Autodesk Inventor part; units mm, degrees
(part 10 of 10)
  spline S24 degree 5 poles (-3.4199, 4.4832) (-3.4186, 4.4814) (-3.4221, 4.4861) (-3.4215, 4.4854) (-3.4253, 4.4909) (-3.428, 4.4951) (-3.4307, 4.4992) (-3.4365, 4.5085) (-3.4424, 4.5184) (-3.4458, 4.5243) (-3.4538, 4.5385) (-3.4613, 4.5527) (-3.4656, 4.5609) (-3.4749, 4.5792) (-3.4837, 4.5978) (-3.4884, 4.608) (-3.4985, 4.6304) (-3.508, 4.6531) (-3.513, 4.6653) (-3.5233, 4.6916) (-3.5331, 4.7182) (-3.5382, 4.7323) (-3.5485, 4.7624) (-3.5582, 4.7926) (-3.5631, 4.8086) (-3.573, 4.8422) (-3.5823, 4.8761) (-3.587, 4.8938) (-3.5964, 4.9308) (-3.6049, 4.9679) (-3.6092, 4.9872) (-3.6176, 5.0274) (-3.6253, 5.0677) (-3.629, 5.0885) (-3.6363, 5.1317) (-3.6427, 5.175) (-3.6458, 5.1973) (-3.6518, 5.2433) (-3.6568, 5.2893) (-3.6592, 5.313) (-3.6636, 5.3617) (-3.667, 5.4104) (-3.6686, 5.4354) (-3.6712, 5.4865) (-3.673, 5.5377) (-3.6736, 5.5639) (-3.6744, 5.6173) (-3.6742, 5.6708) (-3.6739, 5.6981) (-3.6729, 5.7437) (-3.6712, 5.7892) (-3.6704, 5.8075) (-3.6696, 5.8257) (-3.6686, 5.8439) knots 0 0 0 0 0 0 0.005206 0.005206 0.005206 0.020768 0.020768 0.020768 0.045447 0.045447 0.045447 0.078301 0.078301 0.078301 0.118594 0.118594 0.118594 0.165744 0.165744 0.165744 0.219295 0.219295 0.219295 0.278897 0.278897 0.278897 0.344176 0.344176 0.344176 0.414704 0.414704 0.414704 0.490245 0.490245 0.490245 0.570535 0.570535 0.570535 0.655343 0.655343 0.655343 0.744467 0.744467 0.744467 0.837726 0.837726 0.837726 0.934962 0.934962 0.934962 1 1 1 1 1 1
  spline S25 degree 5 poles (-3.2267, 6.0991) (-3.2141, 6.0927) (-3.2016, 6.0863) (-3.1891, 6.0798) (-3.1559, 6.0624) (-3.123, 6.0445) (-3.1024, 6.0333) (-3.0623, 6.0108) (-3.0225, 5.9876) (-3.003, 5.9761) (-2.965, 5.9532) (-2.9273, 5.9297) (-2.9089, 5.9181) (-2.873, 5.8949) (-2.8375, 5.8711) (-2.8201, 5.8593) (-2.7864, 5.836) (-2.7531, 5.8121) (-2.7369, 5.8003) (-2.7054, 5.777) (-2.6743, 5.7531) (-2.6593, 5.7413) (-2.63, 5.7181) (-2.6012, 5.6945) (-2.5873, 5.6828) (-2.5603, 5.6599) (-2.5338, 5.6366) (-2.521, 5.6251) (-2.4964, 5.6027) (-2.4721, 5.5799) (-2.4605, 5.5688) (-2.4382, 5.547) (-2.4164, 5.5249) (-2.4059, 5.5142) (-2.386, 5.4933) (-2.3665, 5.472) (-2.3572, 5.4618) (-2.3396, 5.442) (-2.3223, 5.4218) (-2.3142, 5.4122) (-2.299, 5.3937) (-2.2841, 5.375) (-2.2771, 5.366) (-2.2642, 5.3492) (-2.2516, 5.3321) (-2.2458, 5.3241) (-2.2353, 5.3091) (-2.225, 5.294) (-2.2204, 5.2869) (-2.2121, 5.2741) (-2.2041, 5.2612) (-2.2005, 5.2554) (-2.1945, 5.2452) (-2.1886, 5.2348) (-2.1862, 5.2304) (-2.1823, 5.2232) (-2.1786, 5.216) (-2.1771, 5.213) (-2.1743, 5.2073) (-2.1712, 5.2005) (-2.1718, 5.2008) (-2.1651, 5.1878) (-2.1723, 5.2027) knots 0 0 0 0 0 0 0.049689 0.049689 0.049689 0.132369 0.132369 0.132369 0.212233 0.212233 0.212233 0.289188 0.289188 0.289188 0.363131 0.363131 0.363131 0.433949 0.433949 0.433949 0.501515 0.501515 0.501515 0.565688 0.565688 0.565688 0.626312 0.626312 0.626312 0.683208 0.683208 0.683208 0.736174 0.736174 0.736174 0.785106 0.785106 0.785106 0.829714 0.829714 0.829714 0.869672 0.869672 0.869672 0.904603 0.904603 0.904603 0.934334 0.934334 0.934334 0.958417 0.958417 0.958417 0.976245 0.976245 0.976245 0.987326 0.987326 0.987326 1 1 1 1 1 1
  spline S26 degree 5 poles (-0.7202, 5.5925) (-0.7199, 5.5903) (-0.7206, 5.5961) (-0.7204, 5.5952) (-0.721, 5.6019) (-0.7212, 5.6069) (-0.7214, 5.6117) (-0.7218, 5.6228) (-0.722, 5.6343) (-0.722, 5.6411) (-0.7218, 5.6573) (-0.7213, 5.6734) (-0.7209, 5.6826) (-0.7197, 5.7031) (-0.7181, 5.7236) (-0.7171, 5.7349) (-0.7145, 5.7593) (-0.7115, 5.7837) (-0.7097, 5.7968) (-0.7055, 5.8247) (-0.7007, 5.8526) (-0.698, 5.8674) (-0.6919, 5.8986) (-0.6851, 5.9296) (-0.6814, 5.9459) (-0.6732, 5.98) (-0.6644, 6.014) (-0.6595, 6.0316) (-0.6492, 6.0683) (-0.638, 6.1048) (-0.632, 6.1237) (-0.6193, 6.1627) (-0.6057, 6.2014) (-0.5985, 6.2213) (-0.5833, 6.2623) (-0.5672, 6.303) (-0.5587, 6.3239) (-0.5409, 6.3667) (-0.5222, 6.4091) (-0.5124, 6.4308) (-0.4919, 6.4751) (-0.4706, 6.5191) (-0.4594, 6.5415) (-0.4361, 6.5871) (-0.412, 6.6323) (-0.3995, 6.6552) (-0.3734, 6.702) (-0.3465, 6.7482) (-0.3326, 6.7717) (-0.309, 6.8106) (-0.2848, 6.8492) (-0.275, 6.8646) (-0.2651, 6.88) (-0.2551, 6.8953) knots 0 0 0 0 0 0 0.005206 0.005206 0.005206 0.020768 0.020768 0.020768 0.045447 0.045447 0.045447 0.078301 0.078301 0.078301 0.118594 0.118594 0.118594 0.165744 0.165744 0.165744 0.219295 0.219295 0.219295 0.278897 0.278897 0.278897 0.344176 0.344176 0.344176 0.414704 0.414704 0.414704 0.490245 0.490245 0.490245 0.570535 0.570535 0.570535 0.655343 0.655343 0.655343 0.744467 0.744467 0.744467 0.837726 0.837726 0.837726 0.934962 0.934962 0.934962 1 1 1 1 1 1
  spline S27 degree 5 poles (0.2551, 6.8953) (0.2628, 6.8835) (0.2704, 6.8717) (0.278, 6.8598) (0.2981, 6.8281) (0.3177, 6.7962) (0.3298, 6.7762) (0.3534, 6.7366) (0.3763, 6.6967) (0.3874, 6.677) (0.4089, 6.6381) (0.4298, 6.5989) (0.4399, 6.5796) (0.4594, 6.5416) (0.4782, 6.5033) (0.4873, 6.4844) (0.5049, 6.4473) (0.5218, 6.41) (0.5299, 6.3917) (0.5455, 6.3557) (0.5605, 6.3195) (0.5677, 6.3018) (0.5814, 6.2671) (0.5945, 6.2321) (0.6008, 6.2151) (0.6127, 6.1818) (0.624, 6.1483) (0.6293, 6.132) (0.6394, 6.1003) (0.649, 6.0684) (0.6535, 6.053) (0.6619, 6.023) (0.6698, 5.9929) (0.6735, 5.9784) (0.6803, 5.9503) (0.6866, 5.9222) (0.6895, 5.9086) (0.6948, 5.8827) (0.6997, 5.8566) (0.7019, 5.8442) (0.7059, 5.8206) (0.7094, 5.7969) (0.711, 5.7857) (0.7137, 5.7646) (0.7161, 5.7436) (0.7171, 5.7337) (0.7188, 5.7155) (0.7201, 5.6972) (0.7206, 5.6888) (0.7213, 5.6736) (0.7218, 5.6584) (0.722, 5.6515) (0.7221, 5.6397) (0.722, 5.6278) (0.7219, 5.6228) (0.7217, 5.6145) (0.7213, 5.6064) (0.7211, 5.6031) (0.7206, 5.5968) (0.7199, 5.5894) (0.7195, 5.5899) (0.7189, 5.5753) (0.7201, 5.5919) knots 0 0 0 0 0 0 0.049689 0.049689 0.049689 0.132369 0.132369 0.132369 0.212233 0.212233 0.212233 0.289188 0.289188 0.289188 0.363131 0.363131 0.363131 0.433949 0.433949 0.433949 0.501515 0.501515 0.501515 0.565688 0.565688 0.565688 0.626312 0.626312 0.626312 0.683208 0.683208 0.683208 0.736174 0.736174 0.736174 0.785106 0.785106 0.785106 0.829714 0.829714 0.829714 0.869672 0.869672 0.869672 0.904603 0.904603 0.904603 0.934334 0.934334 0.934334 0.958417 0.958417 0.958417 0.976245 0.976245 0.976245 0.987326 0.987326 0.987326 1 1 1 1 1 1
  spline S28 degree 5 poles (2.1726, 5.2033) (2.1717, 5.2013) (2.174, 5.2067) (2.1737, 5.2058) (2.1766, 5.2119) (2.1789, 5.2163) (2.1811, 5.2206) (2.1863, 5.2304) (2.1919, 5.2404) (2.1953, 5.2463) (2.2035, 5.2603) (2.2121, 5.2739) (2.217, 5.2817) (2.2283, 5.2989) (2.2399, 5.3158) (2.2465, 5.3251) (2.2608, 5.345) (2.2757, 5.3645) (2.2838, 5.375) (2.3014, 5.3971) (2.3195, 5.4189) (2.3292, 5.4303) (2.3501, 5.4543) (2.3715, 5.4778) (2.3829, 5.49) (2.407, 5.5155) (2.4316, 5.5404) (2.4446, 5.5533) (2.472, 5.5799) (2.4999, 5.6059) (2.5145, 5.6193) (2.545, 5.6467) (2.5761, 5.6734) (2.5923, 5.6871) (2.626, 5.715) (2.6603, 5.7422) (2.6781, 5.756) (2.7149, 5.7842) (2.7523, 5.8116) (2.7716, 5.8255) (2.8116, 5.8536) (2.852, 5.8809) (2.8729, 5.8948) (2.9158, 5.9226) (2.9593, 5.9497) (2.9817, 5.9634) (3.0276, 5.9908) (3.074, 6.0174) (3.0978, 6.0307) (3.1377, 6.0526) (3.178, 6.074) (3.1942, 6.0824) (3.2104, 6.0908) (3.2267, 6.0991) knots 0 0 0 0 0 0 0.005206 0.005206 0.005206 0.020768 0.020768 0.020768 0.045447 0.045447 0.045447 0.078301 0.078301 0.078301 0.118594 0.118594 0.118594 0.165744 0.165744 0.165744 0.219295 0.219295 0.219295 0.278897 0.278897 0.278897 0.344176 0.344176 0.344176 0.414704 0.414704 0.414704 0.490245 0.490245 0.490245 0.570535 0.570535 0.570535 0.655343 0.655343 0.655343 0.744467 0.744467 0.744467 0.837726 0.837726 0.837726 0.934962 0.934962 0.934962 1 1 1 1 1 1
  spline S29 degree 5 poles (3.6686, 5.8439) (3.6693, 5.8299) (3.67, 5.8158) (3.6707, 5.8018) (3.6722, 5.7643) (3.6733, 5.7268) (3.6737, 5.7034) (3.6743, 5.6574) (3.6742, 5.6114) (3.674, 5.5888) (3.6732, 5.5444) (3.6717, 5.5) (3.6707, 5.4782) (3.6686, 5.4355) (3.6658, 5.3929) (3.6643, 5.372) (3.6609, 5.3311) (3.6569, 5.2903) (3.6548, 5.2704) (3.6503, 5.2315) (3.6452, 5.1926) (3.6425, 5.1736) (3.637, 5.1367) (3.6309, 5.0999) (3.6278, 5.082) (3.6215, 5.0473) (3.6145, 5.0126) (3.611, 4.9958) (3.6039, 4.9633) (3.5963, 4.9309) (3.5924, 4.9153) (3.5848, 4.8851) (3.5765, 4.8551) (3.5725, 4.8407) (3.5643, 4.813) (3.5557, 4.7854) (3.5515, 4.7722) (3.5431, 4.7471) (3.5343, 4.7221) (3.53, 4.7103) (3.5216, 4.6878) (3.5128, 4.6655) (3.5086, 4.655) (3.5004, 4.6355) (3.4919, 4.616) (3.4879, 4.607) (3.4802, 4.5904) (3.4722, 4.5739) (3.4684, 4.5664) (3.4615, 4.5528) (3.4543, 4.5394) (3.451, 4.5334) (3.4452, 4.5231) (3.4392, 4.5128) (3.4366, 4.5085) (3.4323, 4.5015) (3.4279, 4.4947) (3.426, 4.4919) (3.4225, 4.4867) (3.4181, 4.4806) (3.4181, 4.4812) (3.4102, 4.4689) (3.4195, 4.4827) knots 0 0 0 0 0 0 0.049689 0.049689 0.049689 0.132369 0.132369 0.132369 0.212233 0.212233 0.212233 0.289188 0.289188 0.289188 0.363131 0.363131 0.363131 0.433949 0.433949 0.433949 0.501515 0.501515 0.501515 0.565688 0.565688 0.565688 0.626312 0.626312 0.626312 0.683208 0.683208 0.683208 0.736174 0.736174 0.736174 0.785106 0.785106 0.785106 0.829714 0.829714 0.829714 0.869672 0.869672 0.869672 0.904603 0.904603 0.904603 0.934334 0.934334 0.934334 0.958417 0.958417 0.958417 0.976245 0.976245 0.976245 0.987326 0.987326 0.987326 1 1 1 1 1 1
  spline S30 degree 5 poles (4.4832, 3.4199) (4.4814, 3.4186) (4.4861, 3.4221) (4.4854, 3.4215) (4.4909, 3.4253) (4.4951, 3.428) (4.4992, 3.4307) (4.5085, 3.4365) (4.5184, 3.4424) (4.5243, 3.4458) (4.5385, 3.4538) (4.5527, 3.4613) (4.5609, 3.4656) (4.5792, 3.4749) (4.5978, 3.4837) (4.608, 3.4884) (4.6304, 3.4985) (4.6531, 3.508) (4.6653, 3.513) (4.6916, 3.5233) (4.7182, 3.5331) (4.7323, 3.5382) (4.7624, 3.5485) (4.7926, 3.5582) (4.8086, 3.5631) (4.8422, 3.573) (4.8761, 3.5823) (4.8938, 3.587) (4.9308, 3.5964) (4.9679, 3.6049) (4.9872, 3.6092) (5.0274, 3.6176) (5.0677, 3.6253) (5.0885, 3.629) (5.1317, 3.6363) (5.175, 3.6427) (5.1973, 3.6458) (5.2433, 3.6518) (5.2893, 3.6568) (5.313, 3.6592) (5.3617, 3.6636) (5.4104, 3.667) (5.4354, 3.6686) (5.4865, 3.6712) (5.5377, 3.673) (5.5639, 3.6736) (5.6173, 3.6744) (5.6708, 3.6742) (5.6981, 3.6739) (5.7437, 3.6729) (5.7892, 3.6712) (5.8075, 3.6704) (5.8257, 3.6696) (5.8439, 3.6686) knots 0 0 0 0 0 0 0.005206 0.005206 0.005206 0.020768 0.020768 0.020768 0.045447 0.045447 0.045447 0.078301 0.078301 0.078301 0.118594 0.118594 0.118594 0.165744 0.165744 0.165744 0.219295 0.219295 0.219295 0.278897 0.278897 0.278897 0.344176 0.344176 0.344176 0.414704 0.414704 0.414704 0.490245 0.490245 0.490245 0.570535 0.570535 0.570535 0.655343 0.655343 0.655343 0.744467 0.744467 0.744467 0.837726 0.837726 0.837726 0.934962 0.934962 0.934962 1 1 1 1 1 1
  spline S31 degree 5 poles (6.0991, 3.2267) (6.0927, 3.2141) (6.0863, 3.2016) (6.0798, 3.1891) (6.0624, 3.1559) (6.0445, 3.123) (6.0333, 3.1024) (6.0108, 3.0623) (5.9876, 3.0225) (5.9761, 3.003) (5.9532, 2.965) (5.9297, 2.9273) (5.9181, 2.9089) (5.8949, 2.873) (5.8711, 2.8375) (5.8593, 2.8201) (5.836, 2.7864) (5.8121, 2.7531) (5.8003, 2.7369) (5.777, 2.7054) (5.7531, 2.6743) (5.7413, 2.6593) (5.7181, 2.63) (5.6945, 2.6012) (5.6828, 2.5873) (5.6599, 2.5603) (5.6366, 2.5338) (5.6251, 2.521) (5.6027, 2.4964) (5.5799, 2.4721) (5.5688, 2.4605) (5.547, 2.4382) (5.5249, 2.4164) (5.5142, 2.4059) (5.4933, 2.386) (5.472, 2.3665) (5.4618, 2.3572) (5.442, 2.3396) (5.4218, 2.3223) (5.4122, 2.3142) (5.3937, 2.299) (5.375, 2.2841) (5.366, 2.2771) (5.3492, 2.2642) (5.3321, 2.2516) (5.3241, 2.2458) (5.3091, 2.2353) (5.294, 2.225) (5.2869, 2.2204) (5.2741, 2.2121) (5.2612, 2.2041) (5.2554, 2.2005) (5.2452, 2.1945) (5.2348, 2.1886) (5.2304, 2.1862) (5.2232, 2.1823) (5.216, 2.1786) (5.213, 2.1771) (5.2073, 2.1743) (5.2005, 2.1712) (5.2008, 2.1718) (5.1878, 2.1651) (5.2027, 2.1723) knots 0 0 0 0 0 0 0.049689 0.049689 0.049689 0.132369 0.132369 0.132369 0.212233 0.212233 0.212233 0.289188 0.289188 0.289188 0.363131 0.363131 0.363131 0.433949 0.433949 0.433949 0.501515 0.501515 0.501515 0.565688 0.565688 0.565688 0.626312 0.626312 0.626312 0.683208 0.683208 0.683208 0.736174 0.736174 0.736174 0.785106 0.785106 0.785106 0.829714 0.829714 0.829714 0.869672 0.869672 0.869672 0.904603 0.904603 0.904603 0.934334 0.934334 0.934334 0.958417 0.958417 0.958417 0.976245 0.976245 0.976245 0.987326 0.987326 0.987326 1 1 1 1 1 1
  spline S32 degree 5 poles (5.5925, 0.7202) (5.5903, 0.7199) (5.5961, 0.7206) (5.5952, 0.7204) (5.6019, 0.721) (5.6069, 0.7212) (5.6117, 0.7214) (5.6228, 0.7218) (5.6343, 0.722) (5.6411, 0.722) (5.6573, 0.7218) (5.6734, 0.7213) (5.6826, 0.7209) (5.7031, 0.7197) (5.7236, 0.7181) (5.7349, 0.7171) (5.7593, 0.7145) (5.7837, 0.7115) (5.7968, 0.7097) (5.8247, 0.7055) (5.8526, 0.7007) (5.8674, 0.698) (5.8986, 0.6919) (5.9296, 0.6851) (5.9459, 0.6814) (5.98, 0.6732) (6.014, 0.6644) (6.0316, 0.6595) (6.0683, 0.6492) (6.1048, 0.638) (6.1237, 0.632) (6.1627, 0.6193) (6.2014, 0.6057) (6.2213, 0.5985) (6.2623, 0.5833) (6.303, 0.5672) (6.3239, 0.5587) (6.3667, 0.5409) (6.4091, 0.5222) (6.4308, 0.5124) (6.4751, 0.4919) (6.5191, 0.4706) (6.5415, 0.4594) (6.5871, 0.4361) (6.6323, 0.412) (6.6552, 0.3995) (6.702, 0.3734) (6.7482, 0.3465) (6.7717, 0.3326) (6.8106, 0.309) (6.8492, 0.2848) (6.8646, 0.275) (6.88, 0.2651) (6.8953, 0.2551) knots 0 0 0 0 0 0 0.005206 0.005206 0.005206 0.020768 0.020768 0.020768 0.045447 0.045447 0.045447 0.078301 0.078301 0.078301 0.118594 0.118594 0.118594 0.165744 0.165744 0.165744 0.219295 0.219295 0.219295 0.278897 0.278897 0.278897 0.344176 0.344176 0.344176 0.414704 0.414704 0.414704 0.490245 0.490245 0.490245 0.570535 0.570535 0.570535 0.655343 0.655343 0.655343 0.744467 0.744467 0.744467 0.837726 0.837726 0.837726 0.934962 0.934962 0.934962 1 1 1 1 1 1
  spline S33 degree 5 poles (6.8953, -0.2551) (6.8835, -0.2628) (6.8717, -0.2704) (6.8598, -0.278) (6.8281, -0.2981) (6.7962, -0.3177) (6.7762, -0.3298) (6.7366, -0.3534) (6.6967, -0.3763) (6.677, -0.3874) (6.6381, -0.4089) (6.5989, -0.4298) (6.5796, -0.4399) (6.5416, -0.4594) (6.5033, -0.4782) (6.4844, -0.4873) (6.4473, -0.5049) (6.41, -0.5218) (6.3917, -0.5299) (6.3557, -0.5455) (6.3195, -0.5605) (6.3018, -0.5677) (6.2671, -0.5814) (6.2321, -0.5945) (6.2151, -0.6008) (6.1818, -0.6127) (6.1483, -0.624) (6.132, -0.6293) (6.1003, -0.6394) (6.0684, -0.649) (6.053, -0.6535) (6.023, -0.6619) (5.9929, -0.6698) (5.9784, -0.6735) (5.9503, -0.6803) (5.9222, -0.6866) (5.9086, -0.6895) (5.8827, -0.6948) (5.8566, -0.6997) (5.8442, -0.7019) (5.8206, -0.7059) (5.7969, -0.7094) (5.7857, -0.711) (5.7646, -0.7137) (5.7436, -0.7161) (5.7337, -0.7171) (5.7155, -0.7188) (5.6972, -0.7201) (5.6888, -0.7206) (5.6736, -0.7213) (5.6584, -0.7218) (5.6515, -0.722) (5.6397, -0.7221) (5.6278, -0.722) (5.6228, -0.7219) (5.6145, -0.7217) (5.6064, -0.7213) (5.6031, -0.7211) (5.5968, -0.7206) (5.5894, -0.7199) (5.5899, -0.7195) (5.5753, -0.7189) (5.5919, -0.7201) knots 0 0 0 0 0 0 0.049689 0.049689 0.049689 0.132369 0.132369 0.132369 0.212233 0.212233 0.212233 0.289188 0.289188 0.289188 0.363131 0.363131 0.363131 0.433949 0.433949 0.433949 0.501515 0.501515 0.501515 0.565688 0.565688 0.565688 0.626312 0.626312 0.626312 0.683208 0.683208 0.683208 0.736174 0.736174 0.736174 0.785106 0.785106 0.785106 0.829714 0.829714 0.829714 0.869672 0.869672 0.869672 0.904603 0.904603 0.904603 0.934334 0.934334 0.934334 0.958417 0.958417 0.958417 0.976245 0.976245 0.976245 0.987326 0.987326 0.987326 1 1 1 1 1 1
  spline S34 degree 5 poles (5.2033, -2.1726) (5.2013, -2.1717) (5.2067, -2.174) (5.2058, -2.1737) (5.2119, -2.1766) (5.2163, -2.1789) (5.2206, -2.1811) (5.2304, -2.1863) (5.2404, -2.1919) (5.2463, -2.1953) (5.2603, -2.2035) (5.2739, -2.2121) (5.2817, -2.217) (5.2989, -2.2283) (5.3158, -2.2399) (5.3251, -2.2465) (5.345, -2.2608) (5.3645, -2.2757) (5.375, -2.2838) (5.3971, -2.3014) (5.4189, -2.3195) (5.4303, -2.3292) (5.4543, -2.3501) (5.4778, -2.3715) (5.49, -2.3829) (5.5155, -2.407) (5.5404, -2.4316) (5.5533, -2.4446) (5.5799, -2.472) (5.6059, -2.4999) (5.6193, -2.5145) (5.6467, -2.545) (5.6734, -2.5761) (5.6871, -2.5923) (5.715, -2.626) (5.7422, -2.6603) (5.756, -2.6781) (5.7842, -2.7149) (5.8116, -2.7523) (5.8255, -2.7716) (5.8536, -2.8116) (5.8809, -2.852) (5.8948, -2.8729) (5.9226, -2.9158) (5.9497, -2.9593) (5.9634, -2.9817) (5.9908, -3.0276) (6.0174, -3.074) (6.0307, -3.0978) (6.0526, -3.1377) (6.074, -3.178) (6.0824, -3.1942) (6.0908, -3.2104) (6.0991, -3.2267) knots 0 0 0 0 0 0 0.005206 0.005206 0.005206 0.020768 0.020768 0.020768 0.045447 0.045447 0.045447 0.078301 0.078301 0.078301 0.118594 0.118594 0.118594 0.165744 0.165744 0.165744 0.219295 0.219295 0.219295 0.278897 0.278897 0.278897 0.344176 0.344176 0.344176 0.414704 0.414704 0.414704 0.490245 0.490245 0.490245 0.570535 0.570535 0.570535 0.655343 0.655343 0.655343 0.744467 0.744467 0.744467 0.837726 0.837726 0.837726 0.934962 0.934962 0.934962 1 1 1 1 1 1
  spline S35 degree 5 poles (5.8439, -3.6686) (5.8257, -3.6696) (5.8075, -3.6704) (5.7892, -3.6712) (5.7437, -3.6729) (5.6981, -3.6739) (5.6708, -3.6742) (5.6173, -3.6744) (5.5639, -3.6736) (5.5377, -3.673) (5.4865, -3.6712) (5.4354, -3.6686) (5.4104, -3.667) (5.3617, -3.6636) (5.313, -3.6592) (5.2893, -3.6568) (5.2433, -3.6518) (5.1973, -3.6458) (5.175, -3.6427) (5.1317, -3.6363) (5.0885, -3.629) (5.0677, -3.6253) (5.0274, -3.6176) (4.9872, -3.6092) (4.9679, -3.6049) (4.9308, -3.5964) (4.8938, -3.587) (4.8761, -3.5823) (4.8422, -3.573) (4.8086, -3.5631) (4.7926, -3.5582) (4.7624, -3.5485) (4.7323, -3.5382) (4.7182, -3.5331) (4.6916, -3.5233) (4.6653, -3.513) (4.6531, -3.508) (4.6304, -3.4985) (4.608, -3.4884) (4.5978, -3.4837) (4.5792, -3.4749) (4.5609, -3.4656) (4.5527, -3.4613) (4.5385, -3.4538) (4.5243, -3.4458) (4.5184, -3.4424) (4.5085, -3.4365) (4.4992, -3.4307) (4.4951, -3.428) (4.4909, -3.4253) (4.4854, -3.4215) (4.4861, -3.4221) (4.4814, -3.4186) (4.4832, -3.4199) knots 0 0 0 0 0 0 0.065038 0.065038 0.065038 0.162274 0.162274 0.162274 0.255533 0.255533 0.255533 0.344657 0.344657 0.344657 0.429465 0.429465 0.429465 0.509755 0.509755 0.509755 0.585296 0.585296 0.585296 0.655824 0.655824 0.655824 0.721103 0.721103 0.721103 0.780705 0.780705 0.780705 0.834256 0.834256 0.834256 0.881406 0.881406 0.881406 0.921699 0.921699 0.921699 0.954553 0.954553 0.954553 0.979232 0.979232 0.979232 0.994794 0.994794 0.994794 1 1 1 1 1 1
  spline S36 degree 5 poles (3.4199, -4.4832) (3.4186, -4.4814) (3.4221, -4.4861) (3.4215, -4.4854) (3.4253, -4.4909) (3.428, -4.4951) (3.4307, -4.4992) (3.4365, -4.5085) (3.4424, -4.5184) (3.4458, -4.5243) (3.4538, -4.5385) (3.4613, -4.5527) (3.4656, -4.5609) (3.4749, -4.5792) (3.4837, -4.5978) (3.4884, -4.608) (3.4985, -4.6304) (3.508, -4.6531) (3.513, -4.6653) (3.5233, -4.6916) (3.5331, -4.7182) (3.5382, -4.7323) (3.5485, -4.7624) (3.5582, -4.7926) (3.5631, -4.8086) (3.573, -4.8422) (3.5823, -4.8761) (3.587, -4.8938) (3.5964, -4.9308) (3.6049, -4.9679) (3.6092, -4.9872) (3.6176, -5.0274) (3.6253, -5.0677) (3.629, -5.0885) (3.6363, -5.1317) (3.6427, -5.175) (3.6458, -5.1973) (3.6518, -5.2433) (3.6568, -5.2893) (3.6592, -5.313) (3.6636, -5.3617) (3.667, -5.4104) (3.6686, -5.4354) (3.6712, -5.4865) (3.673, -5.5377) (3.6736, -5.5639) (3.6744, -5.6173) (3.6742, -5.6708) (3.6739, -5.6981) (3.6729, -5.7437) (3.6712, -5.7892) (3.6704, -5.8075) (3.6696, -5.8257) (3.6686, -5.8439) knots 0 0 0 0 0 0 0.005206 0.005206 0.005206 0.020768 0.020768 0.020768 0.045447 0.045447 0.045447 0.078301 0.078301 0.078301 0.118594 0.118594 0.118594 0.165744 0.165744 0.165744 0.219295 0.219295 0.219295 0.278897 0.278897 0.278897 0.344176 0.344176 0.344176 0.414704 0.414704 0.414704 0.490245 0.490245 0.490245 0.570535 0.570535 0.570535 0.655343 0.655343 0.655343 0.744467 0.744467 0.744467 0.837726 0.837726 0.837726 0.934962 0.934962 0.934962 1 1 1 1 1 1
  spline S37 degree 5 poles (3.2267, -6.0991) (3.2141, -6.0927) (3.2016, -6.0863) (3.1891, -6.0798) (3.1559, -6.0624) (3.123, -6.0445) (3.1024, -6.0333) (3.0623, -6.0108) (3.0225, -5.9876) (3.003, -5.9761) (2.965, -5.9532) (2.9273, -5.9297) (2.9089, -5.9181) (2.873, -5.8949) (2.8375, -5.8711) (2.8201, -5.8593) (2.7864, -5.836) (2.7531, -5.8121) (2.7369, -5.8003) (2.7054, -5.777) (2.6743, -5.7531) (2.6593, -5.7413) (2.63, -5.7181) (2.6012, -5.6945) (2.5873, -5.6828) (2.5603, -5.6599) (2.5338, -5.6366) (2.521, -5.6251) (2.4964, -5.6027) (2.4721, -5.5799) (2.4605, -5.5688) (2.4382, -5.547) (2.4164, -5.5249) (2.4059, -5.5142) (2.386, -5.4933) (2.3665, -5.472) (2.3572, -5.4618) (2.3396, -5.442) (2.3223, -5.4218) (2.3142, -5.4122) (2.299, -5.3937) (2.2841, -5.375) (2.2771, -5.366) (2.2642, -5.3492) (2.2516, -5.3321) (2.2458, -5.3241) (2.2353, -5.3091) (2.225, -5.294) (2.2204, -5.2869) (2.2121, -5.2741) (2.2041, -5.2612) (2.2005, -5.2554) (2.1945, -5.2452) (2.1886, -5.2348) (2.1862, -5.2304) (2.1823, -5.2232) (2.1786, -5.216) (2.1771, -5.213) (2.1743, -5.2073) (2.1712, -5.2005) (2.1718, -5.2008) (2.1651, -5.1878) (2.1723, -5.2027) knots 0 0 0 0 0 0 0.049689 0.049689 0.049689 0.132369 0.132369 0.132369 0.212233 0.212233 0.212233 0.289188 0.289188 0.289188 0.363131 0.363131 0.363131 0.433949 0.433949 0.433949 0.501515 0.501515 0.501515 0.565688 0.565688 0.565688 0.626312 0.626312 0.626312 0.683208 0.683208 0.683208 0.736174 0.736174 0.736174 0.785106 0.785106 0.785106 0.829714 0.829714 0.829714 0.869672 0.869672 0.869672 0.904603 0.904603 0.904603 0.934334 0.934334 0.934334 0.958417 0.958417 0.958417 0.976245 0.976245 0.976245 0.987326 0.987326 0.987326 1 1 1 1 1 1
  spline S38 degree 5 poles (0.7202, -5.5925) (0.7199, -5.5903) (0.7206, -5.5961) (0.7204, -5.5952) (0.721, -5.6019) (0.7212, -5.6069) (0.7214, -5.6117) (0.7218, -5.6228) (0.722, -5.6343) (0.722, -5.6411) (0.7218, -5.6573) (0.7213, -5.6734) (0.7209, -5.6826) (0.7197, -5.7031) (0.7181, -5.7236) (0.7171, -5.7349) (0.7145, -5.7593) (0.7115, -5.7837) (0.7097, -5.7968) (0.7055, -5.8247) (0.7007, -5.8526) (0.698, -5.8674) (0.6919, -5.8986) (0.6851, -5.9296) (0.6814, -5.9459) (0.6732, -5.98) (0.6644, -6.014) (0.6595, -6.0316) (0.6492, -6.0683) (0.638, -6.1048) (0.632, -6.1237) (0.6193, -6.1627) (0.6057, -6.2014) (0.5985, -6.2213) (0.5833, -6.2623) (0.5672, -6.303) (0.5587, -6.3239) (0.5409, -6.3667) (0.5222, -6.4091) (0.5124, -6.4308) (0.4919, -6.4751) (0.4706, -6.5191) (0.4594, -6.5415) (0.4361, -6.5871) (0.412, -6.6323) (0.3995, -6.6552) (0.3734, -6.702) (0.3465, -6.7482) (0.3326, -6.7717) (0.309, -6.8106) (0.2848, -6.8492) (0.275, -6.8646) (0.2651, -6.88) (0.2551, -6.8953) knots 0 0 0 0 0 0 0.005206 0.005206 0.005206 0.020768 0.020768 0.020768 0.045447 0.045447 0.045447 0.078301 0.078301 0.078301 0.118594 0.118594 0.118594 0.165744 0.165744 0.165744 0.219295 0.219295 0.219295 0.278897 0.278897 0.278897 0.344176 0.344176 0.344176 0.414704 0.414704 0.414704 0.490245 0.490245 0.490245 0.570535 0.570535 0.570535 0.655343 0.655343 0.655343 0.744467 0.744467 0.744467 0.837726 0.837726 0.837726 0.934962 0.934962 0.934962 1 1 1 1 1 1
  spline S39 degree 5 poles (-0.2551, -6.8953) (-0.2628, -6.8835) (-0.2704, -6.8717) (-0.278, -6.8598) (-0.2981, -6.8281) (-0.3177, -6.7962) (-0.3298, -6.7762) (-0.3534, -6.7366) (-0.3763, -6.6967) (-0.3874, -6.677) (-0.4089, -6.6381) (-0.4298, -6.5989) (-0.4399, -6.5796) (-0.4594, -6.5416) (-0.4782, -6.5033) (-0.4873, -6.4844) (-0.5049, -6.4473) (-0.5218, -6.41) (-0.5299, -6.3917) (-0.5455, -6.3557) (-0.5605, -6.3195) (-0.5677, -6.3018) (-0.5814, -6.2671) (-0.5945, -6.2321) (-0.6008, -6.2151) (-0.6127, -6.1818) (-0.624, -6.1483) (-0.6293, -6.132) (-0.6394, -6.1003) (-0.649, -6.0684) (-0.6535, -6.053) (-0.6619, -6.023) (-0.6698, -5.9929) (-0.6735, -5.9784) (-0.6803, -5.9503) (-0.6866, -5.9222) (-0.6895, -5.9086) (-0.6948, -5.8827) (-0.6997, -5.8566) (-0.7019, -5.8442) (-0.7059, -5.8206) (-0.7094, -5.7969) (-0.711, -5.7857) (-0.7137, -5.7646) (-0.7161, -5.7436) (-0.7171, -5.7337) (-0.7188, -5.7155) (-0.7201, -5.6972) (-0.7206, -5.6888) (-0.7213, -5.6736) (-0.7218, -5.6584) (-0.722, -5.6515) (-0.7221, -5.6397) (-0.722, -5.6278) (-0.7219, -5.6228) (-0.7217, -5.6145) (-0.7213, -5.6064) (-0.7211, -5.6031) (-0.7206, -5.5968) (-0.7199, -5.5894) (-0.7195, -5.5899) (-0.7189, -5.5753) (-0.7201, -5.5919) knots 0 0 0 0 0 0 0.049689 0.049689 0.049689 0.132369 0.132369 0.132369 0.212233 0.212233 0.212233 0.289188 0.289188 0.289188 0.363131 0.363131 0.363131 0.433949 0.433949 0.433949 0.501515 0.501515 0.501515 0.565688 0.565688 0.565688 0.626312 0.626312 0.626312 0.683208 0.683208 0.683208 0.736174 0.736174 0.736174 0.785106 0.785106 0.785106 0.829714 0.829714 0.829714 0.869672 0.869672 0.869672 0.904603 0.904603 0.904603 0.934334 0.934334 0.934334 0.958417 0.958417 0.958417 0.976245 0.976245 0.976245 0.987326 0.987326 0.987326 1 1 1 1 1 1
  spline S40 degree 5 poles (-2.1726, -5.2033) (-2.1717, -5.2013) (-2.174, -5.2067) (-2.1737, -5.2058) (-2.1766, -5.2119) (-2.1789, -5.2163) (-2.1811, -5.2206) (-2.1863, -5.2304) (-2.1919, -5.2404) (-2.1953, -5.2463) (-2.2035, -5.2603) (-2.2121, -5.2739) (-2.217, -5.2817) (-2.2283, -5.2989) (-2.2399, -5.3158) (-2.2465, -5.3251) (-2.2608, -5.345) (-2.2757, -5.3645) (-2.2838, -5.375) (-2.3014, -5.3971) (-2.3195, -5.4189) (-2.3292, -5.4303) (-2.3501, -5.4543) (-2.3715, -5.4778) (-2.3829, -5.49) (-2.407, -5.5155) (-2.4316, -5.5404) (-2.4446, -5.5533) (-2.472, -5.5799) (-2.4999, -5.6059) (-2.5145, -5.6193) (-2.545, -5.6467) (-2.5761, -5.6734) (-2.5923, -5.6871) (-2.626, -5.715) (-2.6603, -5.7422) (-2.6781, -5.756) (-2.7149, -5.7842) (-2.7523, -5.8116) (-2.7716, -5.8255) (-2.8116, -5.8536) (-2.852, -5.8809) (-2.8729, -5.8948) (-2.9158, -5.9226) (-2.9593, -5.9497) (-2.9817, -5.9634) (-3.0276, -5.9908) (-3.074, -6.0174) (-3.0978, -6.0307) (-3.1377, -6.0526) (-3.178, -6.074) (-3.1942, -6.0824) (-3.2104, -6.0908) (-3.2267, -6.0991) knots 0 0 0 0 0 0 0.005206 0.005206 0.005206 0.020768 0.020768 0.020768 0.045447 0.045447 0.045447 0.078301 0.078301 0.078301 0.118594 0.118594 0.118594 0.165744 0.165744 0.165744 0.219295 0.219295 0.219295 0.278897 0.278897 0.278897 0.344176 0.344176 0.344176 0.414704 0.414704 0.414704 0.490245 0.490245 0.490245 0.570535 0.570535 0.570535 0.655343 0.655343 0.655343 0.744467 0.744467 0.744467 0.837726 0.837726 0.837726 0.934962 0.934962 0.934962 1 1 1 1 1 1
  spline S41 degree 5 poles (-3.6686, -5.8439) (-3.6693, -5.8299) (-3.67, -5.8158) (-3.6707, -5.8018) (-3.6722, -5.7643) (-3.6733, -5.7268) (-3.6737, -5.7034) (-3.6743, -5.6574) (-3.6742, -5.6114) (-3.674, -5.5888) (-3.6732, -5.5444) (-3.6717, -5.5) (-3.6707, -5.4782) (-3.6686, -5.4355) (-3.6658, -5.3929) (-3.6643, -5.372) (-3.6609, -5.3311) (-3.6569, -5.2903) (-3.6548, -5.2704) (-3.6503, -5.2315) (-3.6452, -5.1926) (-3.6425, -5.1736) (-3.637, -5.1367) (-3.6309, -5.0999) (-3.6278, -5.082) (-3.6215, -5.0473) (-3.6145, -5.0126) (-3.611, -4.9958) (-3.6039, -4.9633) (-3.5963, -4.9309) (-3.5924, -4.9153) (-3.5848, -4.8851) (-3.5765, -4.8551) (-3.5725, -4.8407) (-3.5643, -4.813) (-3.5557, -4.7854) (-3.5515, -4.7722) (-3.5431, -4.7471) (-3.5343, -4.7221) (-3.53, -4.7103) (-3.5216, -4.6878) (-3.5128, -4.6655) (-3.5086, -4.655) (-3.5004, -4.6355) (-3.4919, -4.616) (-3.4879, -4.607) (-3.4802, -4.5904) (-3.4722, -4.5739) (-3.4684, -4.5664) (-3.4615, -4.5528) (-3.4543, -4.5394) (-3.451, -4.5334) (-3.4452, -4.5231) (-3.4392, -4.5128) (-3.4366, -4.5085) (-3.4323, -4.5015) (-3.4279, -4.4947) (-3.426, -4.4919) (-3.4225, -4.4867) (-3.4181, -4.4806) (-3.4181, -4.4812) (-3.4102, -4.4689) (-3.4195, -4.4827) knots 0 0 0 0 0 0 0.049689 0.049689 0.049689 0.132369 0.132369 0.132369 0.212233 0.212233 0.212233 0.289188 0.289188 0.289188 0.363131 0.363131 0.363131 0.433949 0.433949 0.433949 0.501515 0.501515 0.501515 0.565688 0.565688 0.565688 0.626312 0.626312 0.626312 0.683208 0.683208 0.683208 0.736174 0.736174 0.736174 0.785106 0.785106 0.785106 0.829714 0.829714 0.829714 0.869672 0.869672 0.869672 0.904603 0.904603 0.904603 0.934334 0.934334 0.934334 0.958417 0.958417 0.958417 0.976245 0.976245 0.976245 0.987326 0.987326 0.987326 1 1 1 1 1 1
  spline S42 degree 5 poles (-4.4832, -3.4199) (-4.4814, -3.4186) (-4.4861, -3.4221) (-4.4854, -3.4215) (-4.4909, -3.4253) (-4.4951, -3.428) (-4.4992, -3.4307) (-4.5085, -3.4365) (-4.5184, -3.4424) (-4.5243, -3.4458) (-4.5385, -3.4538) (-4.5527, -3.4613) (-4.5609, -3.4656) (-4.5792, -3.4749) (-4.5978, -3.4837) (-4.608, -3.4884) (-4.6304, -3.4985) (-4.6531, -3.508) (-4.6653, -3.513) (-4.6916, -3.5233) (-4.7182, -3.5331) (-4.7323, -3.5382) (-4.7624, -3.5485) (-4.7926, -3.5582) (-4.8086, -3.5631) (-4.8422, -3.573) (-4.8761, -3.5823) (-4.8938, -3.587) (-4.9308, -3.5964) (-4.9679, -3.6049) (-4.9872, -3.6092) (-5.0274, -3.6176) (-5.0677, -3.6253) (-5.0885, -3.629) (-5.1317, -3.6363) (-5.175, -3.6427) (-5.1973, -3.6458) (-5.2433, -3.6518) (-5.2893, -3.6568) (-5.313, -3.6592) (-5.3617, -3.6636) (-5.4104, -3.667) (-5.4354, -3.6686) (-5.4865, -3.6712) (-5.5377, -3.673) (-5.5639, -3.6736) (-5.6173, -3.6744) (-5.6708, -3.6742) (-5.6981, -3.6739) (-5.7437, -3.6729) (-5.7892, -3.6712) (-5.8075, -3.6704) (-5.8257, -3.6696) (-5.8439, -3.6686) knots 0 0 0 0 0 0 0.005206 0.005206 0.005206 0.020768 0.020768 0.020768 0.045447 0.045447 0.045447 0.078301 0.078301 0.078301 0.118594 0.118594 0.118594 0.165744 0.165744 0.165744 0.219295 0.219295 0.219295 0.278897 0.278897 0.278897 0.344176 0.344176 0.344176 0.414704 0.414704 0.414704 0.490245 0.490245 0.490245 0.570535 0.570535 0.570535 0.655343 0.655343 0.655343 0.744467 0.744467 0.744467 0.837726 0.837726 0.837726 0.934962 0.934962 0.934962 1 1 1 1 1 1
  spline S43 degree 5 poles (-6.0991, -3.2267) (-6.0927, -3.2141) (-6.0863, -3.2016) (-6.0798, -3.1891) (-6.0624, -3.1559) (-6.0445, -3.123) (-6.0333, -3.1024) (-6.0108, -3.0623) (-5.9876, -3.0225) (-5.9761, -3.003) (-5.9532, -2.965) (-5.9297, -2.9273) (-5.9181, -2.9089) (-5.8949, -2.873) (-5.8711, -2.8375) (-5.8593, -2.8201) (-5.836, -2.7864) (-5.8121, -2.7531) (-5.8003, -2.7369) (-5.777, -2.7054) (-5.7531, -2.6743) (-5.7413, -2.6593) (-5.7181, -2.63) (-5.6945, -2.6012) (-5.6828, -2.5873) (-5.6599, -2.5603) (-5.6366, -2.5338) (-5.6251, -2.521) (-5.6027, -2.4964) (-5.5799, -2.4721) (-5.5688, -2.4605) (-5.547, -2.4382) (-5.5249, -2.4164) (-5.5142, -2.4059) (-5.4933, -2.386) (-5.472, -2.3665) (-5.4618, -2.3572) (-5.442, -2.3396) (-5.4218, -2.3223) (-5.4122, -2.3142) (-5.3937, -2.299) (-5.375, -2.2841) (-5.366, -2.2771) (-5.3492, -2.2642) (-5.3321, -2.2516) (-5.3241, -2.2458) (-5.3091, -2.2353) (-5.294, -2.225) (-5.2869, -2.2204) (-5.2741, -2.2121) (-5.2612, -2.2041) (-5.2554, -2.2005) (-5.2452, -2.1945) (-5.2348, -2.1886) (-5.2304, -2.1862) (-5.2232, -2.1823) (-5.216, -2.1786) (-5.213, -2.1771) (-5.2073, -2.1743) (-5.2005, -2.1712) (-5.2008, -2.1718) (-5.1878, -2.1651) (-5.2027, -2.1723) knots 0 0 0 0 0 0 0.049689 0.049689 0.049689 0.132369 0.132369 0.132369 0.212233 0.212233 0.212233 0.289188 0.289188 0.289188 0.363131 0.363131 0.363131 0.433949 0.433949 0.433949 0.501515 0.501515 0.501515 0.565688 0.565688 0.565688 0.626312 0.626312 0.626312 0.683208 0.683208 0.683208 0.736174 0.736174 0.736174 0.785106 0.785106 0.785106 0.829714 0.829714 0.829714 0.869672 0.869672 0.869672 0.904603 0.904603 0.904603 0.934334 0.934334 0.934334 0.958417 0.958417 0.958417 0.976245 0.976245 0.976245 0.987326 0.987326 0.987326 1 1 1 1 1 1
  spline S44 degree 5 poles (-5.5925, -0.7202) (-5.5903, -0.7199) (-5.5961, -0.7206) (-5.5952, -0.7204) (-5.6019, -0.721) (-5.6069, -0.7212) (-5.6117, -0.7214) (-5.6228, -0.7218) (-5.6343, -0.722) (-5.6411, -0.722) (-5.6573, -0.7218) (-5.6734, -0.7213) (-5.6826, -0.7209) (-5.7031, -0.7197) (-5.7236, -0.7181) (-5.7349, -0.7171) (-5.7593, -0.7145) (-5.7837, -0.7115) (-5.7968, -0.7097) (-5.8247, -0.7055) (-5.8526, -0.7007) (-5.8674, -0.698) (-5.8986, -0.6919) (-5.9296, -0.6851) (-5.9459, -0.6814) (-5.98, -0.6732) (-6.014, -0.6644) (-6.0316, -0.6595) (-6.0683, -0.6492) (-6.1048, -0.638) (-6.1237, -0.632) (-6.1627, -0.6193) (-6.2014, -0.6057) (-6.2213, -0.5985) (-6.2623, -0.5833) (-6.303, -0.5672) (-6.3239, -0.5587) (-6.3667, -0.5409) (-6.4091, -0.5222) (-6.4308, -0.5124) (-6.4751, -0.4919) (-6.5191, -0.4706) (-6.5415, -0.4594) (-6.5871, -0.4361) (-6.6323, -0.412) (-6.6552, -0.3995) (-6.702, -0.3734) (-6.7482, -0.3465) (-6.7717, -0.3326) (-6.8106, -0.309) (-6.8492, -0.2848) (-6.8646, -0.275) (-6.88, -0.2651) (-6.8953, -0.2551) knots 0 0 0 0 0 0 0.005206 0.005206 0.005206 0.020768 0.020768 0.020768 0.045447 0.045447 0.045447 0.078301 0.078301 0.078301 0.118594 0.118594 0.118594 0.165744 0.165744 0.165744 0.219295 0.219295 0.219295 0.278897 0.278897 0.278897 0.344176 0.344176 0.344176 0.414704 0.414704 0.414704 0.490245 0.490245 0.490245 0.570535 0.570535 0.570535 0.655343 0.655343 0.655343 0.744467 0.744467 0.744467 0.837726 0.837726 0.837726 0.934962 0.934962 0.934962 1 1 1 1 1 1
  spline S45 degree 5 poles (-6.8953, 0.2551) (-6.8835, 0.2628) (-6.8717, 0.2704) (-6.8598, 0.278) (-6.8281, 0.2981) (-6.7962, 0.3177) (-6.7762, 0.3298) (-6.7366, 0.3534) (-6.6967, 0.3763) (-6.677, 0.3874) (-6.6381, 0.4089) (-6.5989, 0.4298) (-6.5796, 0.4399) (-6.5416, 0.4594) (-6.5033, 0.4782) (-6.4844, 0.4873) (-6.4473, 0.5049) (-6.41, 0.5218) (-6.3917, 0.5299) (-6.3557, 0.5455) (-6.3195, 0.5605) (-6.3018, 0.5677) (-6.2671, 0.5814) (-6.2321, 0.5945) (-6.2151, 0.6008) (-6.1818, 0.6127) (-6.1483, 0.624) (-6.132, 0.6293) (-6.1003, 0.6394) (-6.0684, 0.649) (-6.053, 0.6535) (-6.023, 0.6619) (-5.9929, 0.6698) (-5.9784, 0.6735) (-5.9503, 0.6803) (-5.9222, 0.6866) (-5.9086, 0.6895) (-5.8827, 0.6948) (-5.8566, 0.6997) (-5.8442, 0.7019) (-5.8206, 0.7059) (-5.7969, 0.7094) (-5.7857, 0.711) (-5.7646, 0.7137) (-5.7436, 0.7161) (-5.7337, 0.7171) (-5.7155, 0.7188) (-5.6972, 0.7201) (-5.6888, 0.7206) (-5.6736, 0.7213) (-5.6584, 0.7218) (-5.6515, 0.722) (-5.6397, 0.7221) (-5.6278, 0.722) (-5.6228, 0.7219) (-5.6145, 0.7217) (-5.6064, 0.7213) (-5.6031, 0.7211) (-5.5968, 0.7206) (-5.5894, 0.7199) (-5.5899, 0.7195) (-5.5753, 0.7189) (-5.5919, 0.7201) knots 0 0 0 0 0 0 0.049689 0.049689 0.049689 0.132369 0.132369 0.132369 0.212233 0.212233 0.212233 0.289188 0.289188 0.289188 0.363131 0.363131 0.363131 0.433949 0.433949 0.433949 0.501515 0.501515 0.501515 0.565688 0.565688 0.565688 0.626312 0.626312 0.626312 0.683208 0.683208 0.683208 0.736174 0.736174 0.736174 0.785106 0.785106 0.785106 0.829714 0.829714 0.829714 0.869672 0.869672 0.869672 0.904603 0.904603 0.904603 0.934334 0.934334 0.934334 0.958417 0.958417 0.958417 0.976245 0.976245 0.976245 0.987326 0.987326 0.987326 1 1 1 1 1 1
  spline S46 degree 5 poles (-5.2033, 2.1726) (-5.2013, 2.1717) (-5.2067, 2.174) (-5.2058, 2.1737) (-5.2119, 2.1766) (-5.2163, 2.1789) (-5.2206, 2.1811) (-5.2304, 2.1863) (-5.2404, 2.1919) (-5.2463, 2.1953) (-5.2603, 2.2035) (-5.2739, 2.2121) (-5.2817, 2.217) (-5.2989, 2.2283) (-5.3158, 2.2399) (-5.3251, 2.2465) (-5.345, 2.2608) (-5.3645, 2.2757) (-5.375, 2.2838) (-5.3971, 2.3014) (-5.4189, 2.3195) (-5.4303, 2.3292) (-5.4543, 2.3501) (-5.4778, 2.3715) (-5.49, 2.3829) (-5.5155, 2.407) (-5.5404, 2.4316) (-5.5533, 2.4446) (-5.5799, 2.472) (-5.6059, 2.4999) (-5.6193, 2.5145) (-5.6467, 2.545) (-5.6734, 2.5761) (-5.6871, 2.5923) (-5.715, 2.626) (-5.7422, 2.6603) (-5.756, 2.6781) (-5.7842, 2.7149) (-5.8116, 2.7523) (-5.8255, 2.7716) (-5.8536, 2.8116) (-5.8809, 2.852) (-5.8948, 2.8729) (-5.9226, 2.9158) (-5.9497, 2.9593) (-5.9634, 2.9817) (-5.9908, 3.0276) (-6.0174, 3.074) (-6.0307, 3.0978) (-6.0526, 3.1377) (-6.074, 3.178) (-6.0824, 3.1942) (-6.0908, 3.2104) (-6.0991, 3.2267) knots 0 0 0 0 0 0 0.005206 0.005206 0.005206 0.020768 0.020768 0.020768 0.045447 0.045447 0.045447 0.078301 0.078301 0.078301 0.118594 0.118594 0.118594 0.165744 0.165744 0.165744 0.219295 0.219295 0.219295 0.278897 0.278897 0.278897 0.344176 0.344176 0.344176 0.414704 0.414704 0.414704 0.490245 0.490245 0.490245 0.570535 0.570535 0.570535 0.655343 0.655343 0.655343 0.744467 0.744467 0.744467 0.837726 0.837726 0.837726 0.934962 0.934962 0.934962 1 1 1 1 1 1
  spline S47 degree 5 poles (-5.8439, 3.6686) (-5.8299, 3.6693) (-5.8158, 3.67) (-5.8018, 3.6707) (-5.7643, 3.6722) (-5.7268, 3.6733) (-5.7034, 3.6737) (-5.6574, 3.6743) (-5.6114, 3.6742) (-5.5888, 3.674) (-5.5444, 3.6732) (-5.5, 3.6717) (-5.4782, 3.6707) (-5.4355, 3.6686) (-5.3929, 3.6658) (-5.372, 3.6643) (-5.3311, 3.6609) (-5.2903, 3.6569) (-5.2704, 3.6548) (-5.2315, 3.6503) (-5.1926, 3.6452) (-5.1736, 3.6425) (-5.1367, 3.637) (-5.0999, 3.6309) (-5.082, 3.6278) (-5.0473, 3.6215) (-5.0126, 3.6145) (-4.9958, 3.611) (-4.9633, 3.6039) (-4.9309, 3.5963) (-4.9153, 3.5924) (-4.8851, 3.5848) (-4.8551, 3.5765) (-4.8407, 3.5725) (-4.813, 3.5643) (-4.7854, 3.5557) (-4.7722, 3.5515) (-4.7471, 3.5431) (-4.7221, 3.5343) (-4.7103, 3.53) (-4.6878, 3.5216) (-4.6655, 3.5128) (-4.655, 3.5086) (-4.6355, 3.5004) (-4.616, 3.4919) (-4.607, 3.4879) (-4.5904, 3.4802) (-4.5739, 3.4722) (-4.5664, 3.4684) (-4.5528, 3.4615) (-4.5394, 3.4543) (-4.5334, 3.451) (-4.5231, 3.4452) (-4.5128, 3.4392) (-4.5085, 3.4366) (-4.5015, 3.4323) (-4.4947, 3.4279) (-4.4919, 3.426) (-4.4867, 3.4225) (-4.4806, 3.4181) (-4.4812, 3.4181) (-4.4689, 3.4102) (-4.4827, 3.4195) knots 0 0 0 0 0 0 0.049689 0.049689 0.049689 0.132369 0.132369 0.132369 0.212233 0.212233 0.212233 0.289188 0.289188 0.289188 0.363131 0.363131 0.363131 0.433949 0.433949 0.433949 0.501515 0.501515 0.501515 0.565688 0.565688 0.565688 0.626312 0.626312 0.626312 0.683208 0.683208 0.683208 0.736174 0.736174 0.736174 0.785106 0.785106 0.785106 0.829714 0.829714 0.829714 0.869672 0.869672 0.869672 0.904603 0.904603 0.904603 0.934334 0.934334 0.934334 0.958417 0.958417 0.958417 0.976245 0.976245 0.976245 0.987326 0.987326 0.987326 1 1 1 1 1 1
  dimension "d55" = 0.1
  constraints: 48 end point, 48 point on circle, 24 centre point, 24 concentric, 23 parallel, 120 other
  measures "d55" radial gap between concentric circles of A10 A25
extrude "Extrusion7" cut sketch "Sketch7" against normal up to surface (2 mm away)
sketch "Sketch9" plane through (0, 0, -5) normal (0, 0, -1) x (-1, 0, 0)
  circle A0 centre (0, 0) radius 4.075
  dimension "d62" = 8.15
  constraints: 1 centre point, 1 coincident
  measures "d62" diameter of A0
extrude "Extrusion9" cut sketch "Sketch9" against normal blind 2.6
ref_plane "Work Plane1" through (0, 0, 0) normal (0, 0, 1) x (1, 0, 0)
sketch "Sketch10" plane through (0, 0, 0) normal (0, 0, 1) x (1, 0, 0)
  arc A0 (-15.4415, -1.3095) -> (15.4415, -1.3095) centre (0, -5.5) ccw
  line L0 (11.3137, -16.8137) -> (15.538, -21.038)
  line L1 (11.3137, -16.8137) -> (20.8592, -16.8137) construction
  point P0 (0, 0)
  dimension "d65" = 45
  constraints: 4 end point, 1 horizontal, 1 line through centre, 1 point on circle
  measures "d65" angle of L0 L1
ref_plane "Work Plane2" through (15.538, -21.038, 0) normal (0.7071068, -0.7071068, 0) x (0.7071068, 0.7071068, 0)
sketch "Sketch11" plane through (15.538, -21.038, 0) normal (0.7071068, -0.7071068, 0) x (0.7071068, 0.7071068, 0)
  circle A0 centre (0, 0) radius 1.5
  point P0 (3.8891, 0)
  dimension "d66" = 3
  constraints: 1 centre point, 1 coincident
  measures "d66" diameter of A0
extrude "Extrusion10" cut sketch "Sketch11" against normal blind 8.1
body "Solid1"
